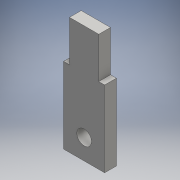
# Autodesk Inventor part: HINGE B
Saved by Autodesk Inventor 2016 (Build 200138000, 138)
## iProperties
Created: 2016-05-27
Part Number: HINGE B
Material: Generic
Document SubType Name: Modeling
Designer: au233088
Density: 1 g/cm^3
Appearance: Default
Author: au233088
Autodesk Inventor part; units mm, degrees
ref_plane "YZ Plane" through (0, 0, 0) normal (1, 0, 0) x (0, 1, 0)
ref_plane "XZ Plane" through (0, 0, 0) normal (0, 1, 0) x (-1, 0, 0)
ref_plane "XY Plane" through (0, 0, 0) normal (0, 0, 1) x (1, 0, 0)
sketch "Sketch3" plane through (0, 0, 0) normal (0, 1, 0) x (-1, 0, 0)
  line L0 (0, 0) -> (-5, 0)
  line L1 (-5, 0) -> (-5, -7)
  line L2 (0, 0) -> (0, -7)
  line L3 (0, -7) -> (1, -7)
  line L4 (1, -7) -> (1, -20)
  line L5 (-5, -7) -> (-6, -7)
  line L6 (-6, -7) -> (-6, -20)
  line L7 (-6, -20) -> (1, -20)
  dimension "d9" = 5
  dimension "d10" = 7
  dimension "d11" = 1
  dimension "d12" = 13
  dimension "d13" = 1
  constraints: 16 end point, 5 perpendicular, 2 horizontal, 1 vertical
  measures "d9" distance of L0.start L0.end
  measures "d10" distance of L0.end L1.end
  measures "d11" distance of L2.end L3.end
  measures "d12" distance of L3.end L4.end
  measures "d13" distance of L1.end L5.end
extrude "Extrusion3" add sketch "Sketch3" along normal blind 2
sketch "Sketch4" plane through (0, 2, 0) normal (0, 1, 0) x (1, 0, 0)
  line L0 (-1, 20) -> (-1, 7) projected
  line L1 (-1, 20) -> (2.5, 20)
  line L2 (6, 20) -> (-1, 20) projected
  line L3 (2.5, 20) -> (2.5, 16.5)
  circle A0 centre (2.5, 16.5) radius 1.25
  point P0 (0, 0)
  dimension "d16" = 3.5
  dimension "d17" = 3.5
  dimension "d18" = 2.5
  constraints: 4 end point, 1 centre point, 1 coincident, 1 midpoint, 1 perpendicular
  measures "d16" distance of L0.start L1.end
  measures "d17" distance of L1.end L3.end
  measures "d18" diameter of A0
extrude "Extrusion4" cut sketch "Sketch4" against normal blind 2
body "Solid2"
